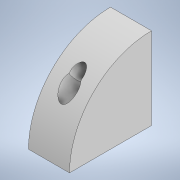
# Autodesk Inventor part: 鋁擠固定器
Saved by Autodesk Inventor 2021 (Build 250183000, 183)
## iProperties
Created: 2023-03-06
Part Number: 鋁擠固定器
Material: 一般
Document SubType Name: Modeling
Designer: brian
Mass: 55.6891 g
Surface Area: 127.827 cm^2
Volume: 55.6891 cm^3
Density: 1 g/cm^3
Appearance: 預設
Author: brian
Autodesk Inventor part; units mm, degrees
ref_plane "YZ Plane" through (0, 0, 0) normal (1, 0, 0) x (0, 1, 0)
ref_plane "XZ Plane" through (0, 0, 0) normal (0, 1, 0) x (-1, 0, 0)
ref_plane "XY Plane" through (0, 0, 0) normal (0, 0, 1) x (1, 0, 0)
sketch "草圖1" plane through (0, 0, 0) normal (1, 0, 0) x (0, 1, 0)
  line L0 (0, 0) -> (0, 65)
  line L1 (0, 65) -> (65, 0)
  line L2 (65, 0) -> (0, 0)
  line L3 (10, 55) -> (0, 55)
  line L4 (55, 10) -> (55, 0)
  line L5 (55, 10) -> (55, 55)
  line L6 (55, 55) -> (10, 55)
  dimension "d0" = 65
  dimension "d1" = 65
  dimension "d20" = 55
  constraints: 14 end point, 5 perpendicular, 4 point on line, 2 vertical
  measures "d0" distance of L0.start L0.end
  measures "d1" distance of L1.end L0.start
  measures "d20" distance between parallel lines of L2 L3
extrude "擠出1" add sketch "草圖1" along normal blind 20 contours L0 L3 L1 L4 L2 | L6 L5 L1
sketch "草圖2" plane through (0, 0, 0) normal (0, -1, 0) x (1, 0, 0)
  line L0 (0, 0) -> (20, 0) projected
  point P0 (10, 30)
  point P1 (10, 0)
  dimension "d4" = 30
  constraints: 1 midpoint, 1 vertical alignment
  measures "d4" distance from line of L0 point (10, 30)
hole "孔1" at (10, 0, 30) direction (0, 1, 0) diameter 4 end through all
sketch "草圖3" plane through (0, 0, 0) normal (0, 0, -1) x (-1, 0, 0)
  line L0 (0, 0) -> (-20, 0) projected
  point P0 (-10, 30)
  point P1 (-10, 0)
  dimension "d12" = 30
  constraints: 1 midpoint, 1 vertical alignment
  measures "d12" distance from line of L0 point (-10, 30)
hole "孔2" at (10, 30, 0) direction (0, 0, 1) diameter 3 end through all
sketch "草圖6" plane through (0, 55, 55) normal (0, 1, 0) x (1, 0, 0)
  circle A0 centre (10, 25) radius 2 projected
  circle A1 centre (10, 25) radius 4
  point P0 (0, 55)
  dimension "d27" = 8
  constraints: 1 centre point, 1 coincident
  measures "d27" diameter of A1
extrude "擠出4" cut sketch "草圖6" against normal blind 50
sketch "草圖7" plane through (0, 0, 55) normal (0, 0, 1) x (1, 0, 0)
  circle A0 centre (10, 30) radius 1.5 projected
  circle A1 centre (10, 30) radius 1.5 projected
  circle A2 centre (10, 30) radius 3
  point P0 (0, 0)
  dimension "d30" = 6
  constraints: 1 centre point, 1 coincident
  measures "d30" diameter of A2
extrude "擠出5" cut sketch "草圖7" against normal blind 50
sketch "草圖8" plane through (20, 0, 0) normal (1, 0, 0) x (0, 0, -1)
  line L0 (0, 0) -> (0, 55) projected
  line L1 (-55, 0) -> (0, 0) projected
  arc A0 (0, 40) -> (-40, 0) centre (0, 0) ccw
  line L2 (-55, 55) -> (-55, 0) projected
  line L3 (-55, 0) -> (0, 0) projected
  line L4 (0, 0) -> (0, 55) projected
  line L5 (0, 55) -> (-55, 55) projected
  dimension "d34" = 40
  constraints: 2 point on circle, 2 point on line, 1 centre point, 1 coincident
  measures "d34" radius of A0
extrude "擠出6" cut sketch "草圖8" against normal through all contours A0 L1 L2 L5 L0
equation "\"d1\" = d0"
